nixal_reprap_XZ_Compatible_robust (Autodesk Fusion 360 design; units mm, degrees)
Autodesk Fusion 360 part; units mm, degrees
sketch "Sketch1" plane through (0, 0, 0) normal (0, 1, 0) x (1, 0, 0)
  circle A0 centre (0, 0) radius 4
  circle A1 centre (21, -2) radius 4
  circle A2 centre (21, -2) radius 13
  circle A3 centre (21, -2) radius 8 construction
  circle A4 centre (29, -2.0036) radius 1.8
  line L0 (21, -2) -> (21, 11) construction
  line L1 (21, -2) -> (34, -2) construction
  line L2 (41, 31) -> (-24, 31)
  line L3 (41, 31) -> (41, -15)
  circle A5 centre (0, 0) radius 10.6
  circle A6 centre (0, 0) radius 13.5
  line L4 (40.8669, 9) -> (-54.1331, 9)
  line L5 (-54.1331, 9) -> (-54.1331, 26)
  line L6 (-54.1331, 26) -> (40.8669, 26)
  line L7 (40.8669, 26) -> (40.8669, 9)
  line L8 (-13.5, 0) -> (-13.5, 9)
  line L9 (34, -2) -> (34, 9)
  line L10 (0, 0) -> (9.5068, -9.5849)
  line L11 (0, 0) -> (7.6248, -11.8995)
  circle A7 centre (21, -2) radius 5.5
  line L12 (13.3463, 2.0311) -> (12.2858, 9)
  line L13 (9.5068, -9.5849) -> (14.0455, -12.9834)
  circle A8 centre (21, 6) radius 1.8
  circle A9 centre (20.9776, -10) radius 1.8
  circle A10 centre (21, -2) radius 12.6491
  circle A11 centre (0, 0) radius 13.0384
  circle A12 centre (21, -2) radius 5.25
  line L14 (-48.7267, 25.5998) -> (-9.6603, 25.5998)
  line L15 (-9.6603, 25.5998) -> (-9.6603, 9.5175)
  line L16 (-9.6603, 9.5175) -> (-48.7267, 9.5175)
  line L17 (-48.7267, 9.5175) -> (-48.7267, 25.5998)
  line L18 (-9.2762, 9) -> (-9.2762, 26)
  line L19 (-48.7267, 18.529) -> (-9.6603, 18.529)
  line L20 (-48.7267, 17.955) -> (-9.6603, 17.955)
  circle A13 centre (0, 0) radius 8
  line L21 (-11.7379, 11.0748) -> (-6.769, 11.0748)
  line L22 (-6.769, 11.0748) -> (-6.769, 13.6262)
  line L23 (-6.769, 13.6262) -> (-11.7379, 13.6262)
  line L24 (-11.7379, 13.6262) -> (-11.7379, 11.0748)
  dimension "d1" = 8
  dimension "d2" = 8
  dimension "d23" = 26
  dimension "d104" = 16
  dimension "d108" = 3.6
  dimension "d134" = 33
  dimension "d136" = 31
  dimension "d137" = 20
  dimension "d138" = 41
  dimension "d139" = 21.2
  dimension "d140" = 27
  dimension "d141" = 17
  dimension "d142" = 95
  dimension "d143" = 5
  dimension "d146" = 11
  dimension "d203" = 3.6
  dimension "d204" = 3.6
  dimension "d211" = 90
  dimension "d225" = 10.5
  dimension "d238" = 16
  dimension "d273" = 21
  dimension "d274" = 2
  constraint coincident A0.centre A5.centre
  constraint concentric A1 A2
  constraint coincident A3
  constraint coincident A2 A0.centre
  constraint vertical L0
  constraint horizontal L1
  constraint horizontal L2
  constraint vertical L3
  constraint concentric A0 A5
  constraint concentric A5 A6
  constraint horizontal L4
  constraint vertical L5
  constraint horizontal L6
  constraint vertical L7
  constraint coincident A6 A0.centre
  constraint coincident L4
  constraint tangent A6 L8
  constraint tangent A2 L9
  constraint coincident A6
  constraint concentric A3 A7
  constraint tangent A6 L12
  constraint coincident A2
  constraint coincident A3 A0.centre
  constraint coincident L0 A0.centre
  constraint concentric A1 A10
  constraint concentric A10 A12
  constraint horizontal L14
  constraint vertical L15
  constraint horizontal L16
  constraint vertical L17
  constraint coincident L6
  constraint perpendicular L6 L18
  constraint coincident L17
  constraint coincident L15
  constraint perpendicular L15 L19
  constraint perpendicular L15 L20
  constraint horizontal L21
  constraint vertical L22
  constraint horizontal L23
  constraint vertical L24
  measures "d1" diameter of A0
  measures "d2" diameter of A1
  measures "d23" diameter of A2
  measures "d104" diameter of A3
  measures "d108" diameter of A4
  measures "d134" distance of A0.centre L2
  measures "d136" distance of A0.centre L2
  measures "d137" distance of A0.centre L3
  measures "d138" distance of A0.centre L3
  measures "d139" diameter of A5
  measures "d140" diameter of A6
  measures "d143" distance of L2 L6
  measures "d146" diameter of A7
  measures "d203" diameter of A8
  measures "d204" diameter of A9
  measures "d211" angle of L4 L8
  measures "d225" diameter of A12
  measures "d238" diameter of A13
extrude "Extrude24" add sketch "Sketch1" along normal blind 70 contours A5 L4 L11 A11 | A5 L10 L11 A11 | A2 A5 L10 A11 | A5 L4 A11 L18 L21 L22 | A6 L10 L11 A11 | A6 L4 L11 A11 | A2 A5 A10 A11 | A2 A6 L10 A11 | A2 A5 L4 A11 | L4 A11 L18 | A6 L4 A11 L18 | A2 A5 A10 A11 | A2 A6 A10 A11 | A5 A10 A11 | A6 L4 A11 L22 | A2 A6 L4 A11 | A6 A11 L18 L21 | A6 L4 L8 | A6 L4 L5 L6 L14 L15 L16 L17 L18 L21 L23 | A2 A6 A10 A11 | A6 A10 A11 | A2 A6 L4 L12 | A2 A6 L4 L6 L7 L18 L22 L23 | A11 L21 L22 | A6 A11 L21 L22 | A6 L18 L21 | A2 A6 L12 A10 | A6 L18 L21 L22 L23 | L15 L18 L21 L23 | A6 L12 A10 | A2 L4 A10 | L15 L21 L23 L24 | L15 L16 L17 L20 L21 L23 L24 | L4 A10 | L15 L17 L19 L20 | L14 L15 L17 L19
extrude "Extrude26" add sketch "Sketch1" along normal blind 70 and the other way blind -54 contours A2 A6 L13 | A2 A6 L4 L13 A10 | A6 L4 L12 A10 | A2 L4 L12 | A2 L4 L12 A10 | A2 L4 L9
sketch "Sketch7" plane through (40.8669, 0, 0) normal (1, 0, 0) x (0, 0, -1)
  line L0 (9, 0) -> (26, 0)
  line L1 (26, 0) -> (26, 70)
  line L2 (26, 70) -> (9, 70)
  line L3 (9, 70) -> (9, 0)
  line L4 (9, 70) -> (26, 0) construction
  line L5 (9, 0) -> (26, 70) construction
  line L6 (17.5, 35) -> (17.5, 57.5) construction
  line L7 (17.5, 35) -> (17.5, 12.5) construction
  circle A0 centre (17.5, 57.5) radius 6
  circle A1 centre (17.5, 12.5) radius 6
  line L8 (23, 50) -> (12, 50)
  line L9 (12, 50) -> (12, 20)
  line L10 (12, 20) -> (23, 20)
  line L11 (23, 20) -> (23, 50)
  line L12 (23, 50) -> (12, 20) construction
  line L13 (12, 50) -> (23, 20) construction
  line L14 (21.801, 47.5) -> (13.199, 47.5)
  line L15 (13.199, 47.5) -> (13.199, 22.5)
  line L16 (13.199, 22.5) -> (21.801, 22.5)
  line L17 (21.801, 22.5) -> (21.801, 47.5)
  line L18 (21.801, 47.5) -> (13.199, 22.5) construction
  line L19 (13.199, 47.5) -> (21.801, 22.5) construction
  line L20 (9, 69.9847) -> (26, 69.9847)
  line L21 (26, 69.9847) -> (26, 0.0176)
  line L22 (26, 0.0176) -> (9, 0.0176)
  line L23 (9, 0.0176) -> (9, 69.9847)
  line L24 (15.7453, 69.9847) -> (18.9725, 69.9847)
  line L25 (17.5, 53.5) -> (15.7453, 53.5)
  line L26 (15.6365, 0.0176) -> (19, 0.0176)
  line L27 (19, 0.0176) -> (19, 8)
  line L28 (19, 8) -> (15.6365, 8)
  line L29 (15.6365, 8) -> (15.6365, 0.0176)
  line L30 (15.7453, 69.9847) -> (18.9725, 69.9847)
  line L31 (18.9725, 62.01) -> (18.9725, 70.9003)
  line L32 (18.9725, 70.9003) -> (15.7453, 70.9003)
  line L33 (15.7453, 70.9003) -> (15.7453, 62.01)
  line L34 (15.7453, 62.01) -> (18.9725, 62.01)
  line L35 (22.75, 40.25) -> (12.25, 40.25)
  line L36 (12.25, 40.25) -> (12.25, 29.75)
  line L37 (12.25, 29.75) -> (22.75, 29.75)
  line L38 (22.75, 29.75) -> (22.75, 40.25)
  line L39 (22.75, 40.25) -> (12.25, 29.75) construction
  line L40 (12.25, 40.25) -> (22.75, 29.75) construction
  dimension "d173" = 22.5
  dimension "d174" = 22.5
  dimension "d175" = 12
  dimension "d176" = 12
  dimension "d179" = 30
  dimension "d180" = 11
  dimension "d195" = 25
  dimension "d275" = 10.5
  dimension "d276" = 10.5
  constraint midpoint L4 origin
  constraint perpendicular L8 L9
  constraint parallel L8 L10
  constraint parallel L9 L11
  constraint horizontal L8
  constraint coincident L12 origin
  constraint coincident L13 origin
  constraint perpendicular L14 L15
  constraint parallel L14 L16
  constraint parallel L15 L17
  constraint horizontal L14
  constraint coincident L18 origin
  constraint coincident L19 origin
  constraint horizontal L20
  constraint vertical L21
  constraint horizontal L22
  constraint vertical L23
  constraint horizontal L24
  constraint vertical L31
  constraint horizontal L25
  constraint vertical L33
  constraint coincident L20 origin
  constraint horizontal L26
  constraint vertical L27
  constraint horizontal L28
  constraint vertical L29
  constraint horizontal L30
  constraint horizontal L32
  constraint perpendicular L31 L34
  constraint coincident L6
  constraint perpendicular L35 L36
  constraint parallel L35 L37
  constraint parallel L36 L38
  constraint horizontal L35
  constraint coincident L39 origin
  constraint coincident L40 origin
  measures "d175" diameter of A0
  measures "d176" diameter of A1
  measures "d195" distance of origin
  measures "d276" distance of origin
extrude "Extrude28" cut sketch "Sketch7" against normal blind 52 contours L8 L9 L10 L11 | L14 L15 L17 L35 | L17 L35 L37 L38 | L15 L17 L35 L37 | L15 L35 L36 L37 | L15 L16 L17 L37
sketch "Sketch8" plane through (0, 0, -9) normal (0, 0, 1) x (1, 0, 0)
  line L0 (-54.1331, 0) -> (-13.5, 0)
  line L1 (-13.5, 0) -> (-13.5, 70)
  line L2 (-13.5, 70) -> (-54.1331, 70)
  line L3 (-54.1331, 70) -> (-54.1331, 0)
  line L4 (-54.1331, 70) -> (-13.5, 0) construction
  line L5 (-13.5, 70) -> (-54.1331, 0) construction
  circle A0 centre (-33.8165, 35) radius 15
  line L6 (-18.3165, 51) -> (-49.3165, 51) construction
  line L7 (-49.3165, 51) -> (-49.3165, 19) construction
  line L8 (-49.3165, 19) -> (-18.3165, 19) construction
  line L9 (-18.3165, 19) -> (-18.3165, 51) construction
  line L10 (-18.3165, 51) -> (-49.3165, 19) construction
  line L11 (-49.3165, 51) -> (-18.3165, 19) construction
  circle A1 centre (-49.3165, 51) radius 1.65
  circle A2 centre (-18.3165, 51) radius 1.65
  circle A3 centre (-49.3165, 19) radius 1.65
  circle A4 centre (-18.3165, 19) radius 1.65
  circle A5 centre (-49.3165, 51) radius 3
  circle A6 centre (-18.3165, 51) radius 3
  circle A7 centre (-18.3165, 19) radius 3
  line L12 (-54.1331, 42.0081) -> (-47.0788, 42.0081)
  line L13 (-26.4517, 0) -> (-26.4517, 21.9325)
  line L14 (-54.1331, 70) -> (-13.5, 70)
  line L15 (-13.5, 70) -> (-13.5, 0)
  line L16 (-13.5, 0) -> (-54.1331, 0)
  line L17 (-54.1331, 0) -> (-54.1331, 70)
  arc A8 (-53.1331, 70) -> (-54.1331, 69) centre (-53.1331, 69) ccw
  line L18 (-54.1331, 70) -> (-13.5, 70)
  line L19 (-13.5, 70) -> (-13.5, 70.2436)
  line L20 (-13.5, 70.2436) -> (-54.1331, 70.2436)
  line L21 (-54.1331, 70.2436) -> (-54.1331, 70)
  circle A9 centre (-49.3165, 19) radius 3
  dimension "d183" = 30
  dimension "d184" = 31
  dimension "d185" = 32
  dimension "d186" = 3.3
  dimension "d187" = 3.3
  dimension "d188" = 3.3
  dimension "d189" = 3.3
  dimension "d190" = 6
  dimension "d191" = 6
  dimension "d192" = 6
  dimension "d202" = 1
  dimension "d250" = 6
  constraint midpoint L4 origin
  constraint perpendicular L6 L7
  constraint parallel L6 L8
  constraint parallel L7 L9
  constraint horizontal L6
  constraint coincident L10 origin
  constraint coincident L11 origin
  constraint concentric A1 A5
  constraint coincident L3 origin
  constraint perpendicular L7 L12
  constraint coincident A0 origin
  constraint perpendicular L8 L13
  constraint horizontal L14
  constraint vertical L15
  constraint horizontal L16
  constraint vertical L17
  constraint coincident L16 origin
  constraint tangent L14 A8
  constraint tangent L17 A8
  constraint coincident L14 origin
  constraint coincident L17 origin
  constraint horizontal L18
  constraint vertical L19
  constraint horizontal L20
  constraint vertical L21
  measures "d183" diameter of A0
  measures "d186" diameter of A1
  measures "d187" diameter of A2
  measures "d188" diameter of A3
  measures "d189" diameter of A4
  measures "d190" diameter of A5
  measures "d191" diameter of A6
  measures "d192" diameter of A7
  measures "d202" radius of A8
  measures "d250" diameter of A9
extrude "Extrude29" cut sketch "Sketch8" against normal blind 40 contours A0 | L2 L3 L14 L17 A8 L18 | A3
extrude "Extrude30" cut sketch "Sketch7" against normal blind 65 contours L14 L15 L17 L35 | L15 L17 L35 L37 | L15 L16 L17 L37
extrude "Extrude31" cut sketch "Sketch8" against normal blind 40 contours A1 | A2 | A4
extrude "Extrude32" cut sketch "Sketch8" against normal blind 9 contours A5 | A6 | A7 | A9
extrude "BELT TUNNEL" add sketch "Sketch7" against normal blind 55 contours L1 L3 A0 A1 L20 L21 L22 L23 L27 L29 L31 L33 | A1 L22 L26 L27 L29 | A0 L20 L24 L30 L31 L33 | A1 L27 L28 L29 | A1 L27 L28 L29 | A0 L31 L33 L34 | A0 L31 L33 L34 | L8 L9 L10 L11 | L14 L15 L17 L35 | L17 L35 L37 L38 | L15 L17 L35 L37 | L15 L35 L36 L37 | L15 L16 L17 L37
extrude "Extrude35" cut sketch "Sketch7" against normal blind 50 contours A1 L22 L26 L27 L29 | A1 L27 L28 L29 picked at (17.3157, 7.501)
extrude "Extrude36" [suppressed]
sketch "Sketch9" plane through (0, 0.0176, 0) normal (0, -1, 0) x (1, 0, 0)
  line L0 (5.6, -9) -> (-5.6, -9)
  circle A0 centre (0, 0) radius 10.6
  line L1 (40.8669, -9) -> (-54.1331, -9)
  arc A1 (-5.6, -9) -> (5.6, -9) centre (0, 0) ccw
extrude "Extrude37" cut sketch "Sketch9" against normal blind 80 contours L0 A0 L1 A1
sketch "Sketch10" plane through (0, 0, -26) normal (0, 0, -1) x (-1, 0, 0)
  circle A0 centre (49.3165, 51) radius 1.65
  circle A1 centre (18.3165, 51) radius 1.65
  circle A2 centre (18.3165, 19) radius 1.65
  arc A3 (54.1331, 69) -> (53.1331, 70) centre (53.1331, 69) ccw
  line L0 (53.1331, 70) -> (-40.8669, 70)
  line L1 (-40.8669, 70) -> (-40.8669, 0)
  line L2 (-40.8669, 0) -> (54.1331, 0)
  line L3 (54.1331, 0) -> (54.1331, 69)
  circle A4 centre (-36.8669, 66) radius 1.65
  circle A5 centre (9.1331, 66) radius 1.65
  circle A6 centre (9.1331, 4.105) radius 1.65
  circle A7 centre (-36.9881, 4.105) radius 1.65
  line L4 (-40.8669, 0.0176) -> (-40.8669, 69.9847)
  circle A8 centre (33.8165, 35) radius 15
  circle A9 centre (49.3165, 19) radius 1.65
  circle A10 centre (-36.8669, 66) radius 2.75
  circle A11 centre (-36.9881, 4.105) radius 2.75
  dimension "d216" = 3.3
  dimension "d217" = 3.3
  dimension "d220" = 3.3
  dimension "d221" = 3.3
  dimension "d243" = 4
  dimension "d259" = 50
  dimension "d260" = 50
  dimension "d268" = 5.5
  dimension "d272" = 5.5
  constraint concentric A4 A10
  constraint concentric A7 A11
  measures "d216" diameter of A4
  measures "d217" diameter of A5
  measures "d220" diameter of A6
  measures "d221" diameter of A7
  measures "d268" diameter of A10
  measures "d272" diameter of A11
extrude "Extrude38" cut sketch "Sketch10" against normal blind 55 contours A4 | A7
sketch "Sketch11" plane through (0, 0, 0) normal (1, 0, 0) x (0, 0, -1)
  line L0 (15.7453, 74.7395) -> (18.9725, 74.7395)
  line L1 (18.9725, 74.7395) -> (18.9725, 53.5)
  line L2 (18.9725, 53.5) -> (15.7453, 53.5)
  line L3 (15.7453, 53.5) -> (15.7453, 74.7395)
  line L4 (15.6365, 8) -> (19.8649, 8)
  line L5 (19.8649, 8) -> (19.8649, -9.5195)
  line L6 (19.8649, -9.5195) -> (15.6365, -9.5195)
  line L7 (15.6365, -9.5195) -> (15.6365, 8)
  constraint horizontal L0
  constraint vertical L1
  constraint horizontal L2
  constraint vertical L3
  constraint horizontal L4
  constraint vertical L5
  constraint horizontal L6
  constraint vertical L7
extrude "opening to tight shafts" cut sketch "Sketch11" along normal blind 85 and the other way blind 14
extrude "Extrude48" cut sketch "Sketch7" against normal blind 55 contours A1 L27 L28 L29 | A1 L27 L28 L29 | A0 L31 L33 L34 | A0 L31 L33 L34
extrude "Extrude49" cut sketch "Sketch7" against normal blind 72 contours L14 L15 L17 L35 | L15 L17 L35 L37 | L15 L16 L17 L37
extrude "Extrude50" [suppressed]
extrude "CUT CHANGES MOTOR TO IDLER" [suppressed]
extrude "Extrude52" cut sketch "Sketch10" against normal blind 17 contours A5 | A6
extrude "Extrude53" cut sketch "Sketch1" along normal blind 8 contours A11 L21 L22 | A6 A11 L21 L22 | A6 L18 L21 L22 L23 | L15 L18 L21 L23 | L15 L21 L23 L24
extrude "Extrude54" cut sketch "Sketch1" along normal blind 80 and the other way blind -61 contours A11 L21 L22 | A6 A11 L21 L22 | A6 L18 L21 L22 L23 | L15 L18 L21 L23 | L15 L21 L23 L24
extrude "Extrude55" cut sketch "Sketch10" along normal blind -45 and the other way blind 15 contours A10 | A11
extrude "Extrude56" cut sketch "Sketch7" against normal blind 54.368 contours L17 L35 L37 L38 | L15 L17 L35 L37 | L15 L35 L36 L37
equation "d173 = ( 45 / 2 ) * 1 mm"
equation "d174 = ( 45 / 2 ) * 1 mm"
